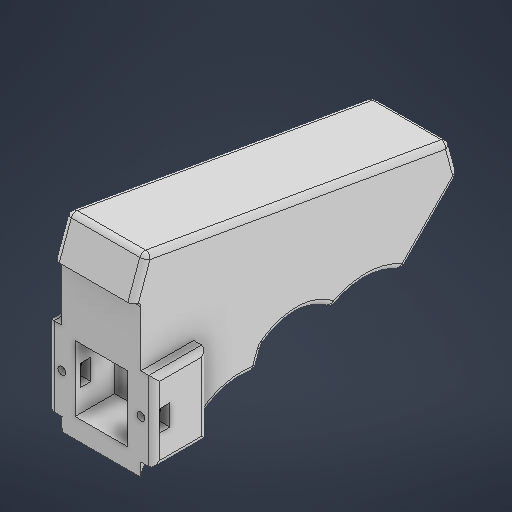
# Autodesk Inventor part: Controller Handle
Saved by Autodesk Inventor 2026.2 (Build 302298010, 298A)
## iProperties
Created: 2026-03-08
Part Number: Controller Handle
Material: Generic
Document SubType Name: Modeling
Designer: barbe
Density: 1 g/cm^3
Appearance: Default
Author: barbe
Autodesk Inventor part; units mm, degrees
ref_plane "YZ Plane" through (0, 0, 0) normal (1, 0, 0) x (0, 1, 0)
ref_plane "XZ Plane" through (0, 0, 0) normal (0, 1, 0) x (-1, 0, 0)
ref_plane "XY Plane" through (0, 0, 0) normal (0, 0, 1) x (1, 0, 0)
sketch "Sketch5" plane through (0, 0, 0) normal (0, 0, 1) x (1, 0, 0)
  line L0 (-10, -12.5) -> (10, -12.5)
  line L1 (10, -12.5) -> (10, 12.5)
  line L2 (10, 12.5) -> (-10, 12.5)
  line L3 (-10, 12.5) -> (-10, -12.5)
  line L4 (-10, -12.5) -> (10, 12.5) construction
  line L5 (10, -12.5) -> (-10, 12.5) construction
  circle A0 centre (15, 0) radius 1.5
  circle A1 centre (-15, 0) radius 1.5
  line L6 (-20, -15) -> (20, -15)
  line L7 (20, -15) -> (20, 15)
  line L8 (20, 15) -> (-20, 15)
  line L9 (-20, 15) -> (-20, -15)
  line L10 (-20, -15) -> (20, 15) construction
  line L11 (20, -15) -> (-20, 15) construction
  line L12 (-20, 0) -> (20, 0)
  line L13 (0, -15) -> (0, 15)
  point P0 (0, 0)
  dimension "d27" = 20
  dimension "d28" = 25
  dimension "d29" = 3
  dimension "d30" = 15
  dimension "d31" = 30
  dimension "d36" = 40
  constraints: 28 end point, 8 midpoint, 4 parallel, 2 centre point, 2 horizontal, 2 perpendicular
  measures "d27" distance of L2.end L1.end
  measures "d28" distance of L1.end L0.end
  measures "d29" diameter of A0
  measures "d30" distance of point (0, 0) A0.centre
  measures "d31" distance of L7.end L6.end
  measures "d36" distance of L7.end L8.end
extrude "Extrusion4" add sketch "Sketch5" along normal blind 20 contours L0 L13 L6 L9 L12 A1 L3 | L0 L1 L12 A0 L7 L6 L13 | L12 A1 L9 L8 L13 L2 L3 | L1 L2 L13 L8 L7 L12 A0
extrude "Extrusion5" add sketch "Sketch5" along normal blind 5 contours L3 L12 L13 L0 | L13 L12 L1 L0 | L3 L2 L13 L12 | L13 L2 L1 L12
extrude "Extrusion6" add sketch "Sketch5" along normal blind 5 contours L12 A1 | A1 L12 | L12 A0 | A0 L12
fillet "Fillet3" radius 2 8 edges at (20, 0, 0) (20, 15, 10) (20, 0, 20) (20, -15, 10) (-20, 0, 0) (-20, -15, 10) (-20, 0, 20) (-20, 15, 10)
sketch "Sketch9" plane through (0, 0, 0) normal (1, 0, 0) x (0, 1, 0)
  line L0 (-12.5, 20) -> (12.5, 20) projected
  line L1 (-36, 20) -> (36, 20)
  arc A0 (36, 20) -> (38, 22) centre (36, 22) ccw
  line L2 (38, 22) -> (38, 23)
  line L3 (15, 0) -> (15, 20) projected
  line L4 (38, 23) -> (52.0954, 17.8697)
  line L5 (38, 23) -> (53, 23) construction
  line L6 (-15, 0) -> (-15, 20) projected
  line L7 (-15, 0) -> (-5, 0) construction
  line L8 (-15, 0) -> (15, 0)
  line L9 (15, 20) -> (15, 0)
  line L10 (-15, 0) -> (-15, 20)
  line L11 (-15, 20) -> (-20, 20)
  arc A1 (-15, 15) -> (-20, 20) centre (-20, 15) ccw
  line L12 (-20, 20) -> (-15, 15) construction
  line L13 (-20, 20) -> (-12.9289, 20) construction
  line L14 (-1.898, -79.3761) -> (19.3152, -100.5893)
  line L15 (19.3152, -100.5893) -> (31.7976, -97.2447)
  line L16 (52.0954, 17.8697) -> (31.7976, -97.2447)
  line L17 (-15, 0) -> (-7.0211, -23.6926)
  arc A2 (-7.0211, -23.6926) -> (-15, 0) centre (-29.9276, -18.217) ccw
  line L18 (-7.0211, -23.6926) -> (0.0266, -26.2577)
  line L19 (-7.0211, -23.6926) -> (0.4789, -23.6926) construction
  line L20 (0.0266, -26.2577) -> (-1.898, -79.3761)
  arc A3 (-0.9357, -52.8168) -> (0.0266, -26.2577) centre (-15.8648, -38.9789) ccw
  arc A4 (-1.898, -79.3761) -> (-0.9357, -52.8168) centre (-22.5407, -65.3311) ccw
  point P0 (0, 0)
  point P1 (0, 20)
  dimension "d46" = 72
  dimension "d47" = 2
  dimension "d48" = 1
  dimension "d60" = 15
  dimension "d61" = 20
  dimension "d73" = 5
  dimension "d74" = 45
  dimension "d79" = 30
  dimension "d81" = 120
  dimension "d91" = 25
  dimension "d94" = 7.5
  dimension "d95" = 20
  dimension "d96" = 26.5765
  constraints: 36 end point, 10 point on circle, 5 centre point, 4 horizontal, 3 collinear, 3 equal length, 3 point on line, 3 tangent, 2 midpoint, 1 perpendicular, 1 vertical
  measures "d46" distance of L1.start L1.end
  measures "d47" radius of A0
  measures "d48" distance of L2.start L2.end
  measures "d60" distance of L2.end L4.end
  measures "d61" angle of L4 L5
  measures "d73" distance of L6.end L11.end
  measures "d74" angle of L12 L13
  measures "d79" distance of L14.start L14.end
  measures "d81" angle of L15 L14
  measures "d91" distance of L6.start L17.end
  measures "d94" distance of L17.end L18.end
  measures "d95" angle of L18 L19
  measures "d96" distance of L18.end A3.start
extrude "Extrusion10" add sketch "Sketch9" along normal mid plane 30 contours L6 A1 L1 | L1 A0 L2 L4 L16 L15 L14 A4 A3 L18 A2 L8 L3
fillet "Fillet4" radius 2 23 edges at (15, -7.6075, -10.7002) (0, 0.0266, -26.2577) (15, -3.4973, -24.9751) (0, -7.0211, -23.6926) (-15, -3.4973, -24.9751) (0, -1.898, -79.3761) (15, 2.4106, -66.2351) (0, -0.9357, -52.8168) (-15, 2.4106, -66.2351) (15, 4.4778, -39.716) (-15, 4.4778, -39.716) (0, 19.3152, -100.5893) (15, 8.7086, -89.9827) (-15, 8.7086, -89.9827) (0, 31.7976, -97.2447) (15, 25.5564, -98.917) (-15, 25.5564, -98.917) (-15, -7.6075, -10.7002) (0, 52.0954, 17.8697) (15, 41.9465, -39.6875) (-15, 41.9465, -39.6875) (-15, 45.0477, 20.4348) (15, 45.0477, 20.4348)
thread "Thread3" size "M3x0.5" class "6H" standard "ANSI Metric M Profile" length 8.001
thread "Thread4" size "M3x0.5" class "6H" standard "ANSI Metric M Profile" length 8.001
sketch "Sketch10" plane through (20, -13, 2) normal (1, 0, 0) x (0, 0, -1)
  line L0 (-16, 0) -> (-16, 26) projected
  line L1 (-16, 13) -> (-12, 13)
  line L2 (-12, 13) -> (-12, 17)
  line L3 (-12, 17) -> (-16, 17)
  line L4 (-16, 17) -> (-16, 13)
  line L5 (-16, 13) -> (-12, 13)
  line L6 (-12, 13) -> (-12, 9)
  line L7 (-12, 9) -> (-16, 9)
  line L8 (-16, 9) -> (-16, 13)
  point P0 (2, 13)
  dimension "d104" = 4
  dimension "d105" = 4
  dimension "d106" = 4
  constraints: 16 end point, 5 equal length, 2 perpendicular, 1 horizontal, 1 midpoint
  measures "d104" distance of L1.start L1.end
  measures "d105" distance of L2.end L1.end
  measures "d106" distance of L1.end L6.end
extrude "Extrusion11" cut sketch "Sketch10" against normal through all
body "Solid2"
